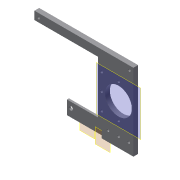
# Autodesk Inventor part: 01_Zeiss_Axiotech_adapterplate_left
Saved by Autodesk Inventor 2019 (Build 230136000, 136)
## iProperties
Created: 2019-05-02
Part Number: 01_Zeiss_Axiotech_adapterplate_left
Material: Generic
Document SubType Name: Modeling
Designer: diederichbenedict
Density: 1 g/cm^3
Appearance: Default
Author: diederichbenedict
Autodesk Inventor part; units mm, degrees
ref_plane "YZ Plane" through (0, 0, 0) normal (1, 0, 0) x (0, 1, 0)
ref_plane "XZ Plane" through (0, 0, 0) normal (0, 1, 0) x (-1, 0, 0)
ref_plane "Work Plane4" through (0, 0, 4) normal (0, 0, 1) x (1, 0, 0)
ref_plane "Work Plane5" through (25.4178, -3.2164, 6.83) normal (0, 0, 1) x (1, 0, 0)
ref_plane "Work Plane6" through (51, 60, 11) normal (0, 0, -1) x (0, 1, 0)
sketch "Sketch9" plane through (51, 60, 11) normal (0, 0, -1) x (0, 1, 0)
  circle A0 centre (0, 25) radius 1.95 construction
  circle A1 centre (-25, 0) radius 1.95 construction
  circle A2 centre (-25, -25) radius 1.95 construction
  circle A3 centre (25, 25) radius 1.95 construction
  circle A4 centre (25, -25) radius 1.95 construction
  circle A5 centre (-25, 25) radius 1.95 construction
  circle A6 centre (25, 0) radius 1.95 construction
  circle A7 centre (0, -25) radius 1.95 construction
  line L0 (-28, 30) -> (-30, 28) construction
  line L1 (-30, 28) -> (-30, -28) construction
  line L2 (-30, -28) -> (-28, -30) construction
  line L3 (-28, -30) -> (28, -30) construction
  line L4 (28, -30) -> (30, -28) construction
  line L5 (30, -28) -> (30, 28) construction
  line L6 (30, 28) -> (28, 30) construction
  line L7 (28, 30) -> (-28, 30) construction
  circle A8 centre (47.5, -118) radius 1.95 construction
  circle A9 centre (47.5, 16) radius 1.95 construction
  line L8 (53.5, -124) -> (41.5, -124)
  line L9 (41.5, -124) -> (41.5, 22)
  line L10 (41.5, 22) -> (53.5, 22)
  line L11 (53.5, 22) -> (53.5, -124)
  circle A10 centre (-60, -51) radius 15 projected
  line L12 (41.5, 22) -> (-60, 22)
  line L13 (-60, 22) -> (-60, -30)
  line L14 (-60, -30) -> (41.5, -30)
  line L15 (41.5, -30) -> (41.5, 22)
  circle A11 centre (47.5, -118) radius 1.95
  circle A12 centre (47.5, 16) radius 1.95
  circle A13 centre (25, -25) radius 2.25
  circle A14 centre (0, -25) radius 2.25
  circle A15 centre (-25, -25) radius 2.25
  circle A16 centre (-25, 0) radius 2.25
  circle A17 centre (25, 0) radius 2.25
  circle A18 centre (0, 0) radius 19.7399
  line L16 (-60, -30) -> (-40, -30)
  line L17 (-40, -30) -> (-40, -80)
  line L18 (-40, -80) -> (-60, -80)
  line L19 (-60, -80) -> (-60, -30)
  point P0 (-60, -51)
  dimension "d32" = 6
  dimension "d33" = 6
  dimension "d34" = 6
  dimension "d35" = 6
  dimension "d36" = 4.5
  dimension "d37" = 4.5
  dimension "d38" = 4.5
  dimension "d39" = 4.5
  dimension "d40" = 4.5
  dimension "d51" = 20
  dimension "d52" = 50
  constraints: 24 end point, 8 centre point, 6 coincident, 6 parallel, 3 horizontal, 3 perpendicular, 2 concentric, 1 point on line
  measures "d32" distance from line of A8.centre L8
  measures "d33" distance from line of L10 A9.centre
  measures "d34" distance from line of L11 A9.centre
  measures "d35" distance from line of L15 A9.centre
  measures "d36" diameter of A13
  measures "d37" diameter of A14
  measures "d38" diameter of A15
  measures "d39" diameter of A16
  measures "d40" diameter of A17
  measures "d51" distance of L17.end L18.end
  measures "d52" distance of L16.end L17.end
extrude "Extrusion8" add sketch "Sketch9" along normal blind 7 contours L8 L9 L10 L11 | L14 L13 L12 L9 | L17 L18 L19 A10 L14 | A10 L19 | A11 | A12 | A13 | A14 | A15 | A16 | A17 picked at (-54.0128, -49.762)
sketch "Sketch10" plane through (51, 60, 4) normal (0, 0, -1) x (-1, 0, 0)
  circle A0 centre (118, 47.5) radius 1.95 projected
  circle A1 centre (-16, 47.5) radius 1.95 projected
  circle A2 centre (-25, 0) radius 1.95 projected
  circle A3 centre (0, -25) radius 1.95 projected
  circle A4 centre (25, -25) radius 1.95 projected
  circle A5 centre (-25, 25) radius 1.95 projected
  circle A6 centre (25, 25) radius 1.95 projected
  circle A7 centre (-25, -25) radius 1.95 projected
  circle A8 centre (0, 25) radius 1.95 projected
  circle A9 centre (25, 0) radius 1.95 projected
  line L0 (-30, -28) -> (-28, -30) projected
  line L1 (-30, 28) -> (-30, -28) projected
  line L2 (-28, 30) -> (-30, 28) projected
  line L3 (28, 30) -> (-28, 30) projected
  line L4 (30, 28) -> (28, 30) projected
  line L5 (30, -28) -> (30, 28) projected
  line L6 (28, -30) -> (30, -28) projected
  line L7 (-28, -30) -> (28, -30) projected
  circle A10 centre (0, 0) radius 19.7399 construction
  line L8 (-22, -60) -> (80, -60) construction
  line L9 (80, -60) -> (80, -40) construction
  line L10 (80, -40) -> (30, -40) construction
  line L11 (30, -40) -> (30, 41.5) construction
  line L12 (30, 41.5) -> (124, 41.5) construction
  line L13 (124, 41.5) -> (124, 53.5) construction
  line L14 (124, 53.5) -> (-22, 53.5) construction
  line L15 (-22, 53.5) -> (-22, -60) construction
  line L16 (-15, -75) -> (15, -75) construction
  line L17 (15, -75) -> (15, -45) construction
  line L18 (15, -45) -> (-15, -45) construction
  line L19 (-15, -45) -> (-15, -75) construction
  line L20 (-22, -60) -> (80, -60) construction
  line L21 (-15, -75) -> (15, -45) construction
  line L22 (15, -75) -> (-15, -45) construction
  point P0 (51, -60)
  point P1 (0, -60)
  point P2 (0, -45)
  point P3 (15.5154, -45.1897)
  dimension "d53" = 30
  dimension "d54" = 30
  constraints: 12 end point, 3 midpoint, 2 parallel, 1 horizontal, 1 perpendicular, 1 point on line
  measures "d53" distance of L18.end L17.end
  measures "d54" distance of L17.end L16.end
hole "Hole2" at (-67, 107.5, 4) at (67, 107.5, 4) at (26, 85, 4) at (26, 60, 4) at (51, 85, 4) at (51, 35, 4) at (26, 35, 4) at (35.4846, 14.8103, 4) at (51, 15, 4) at (66, 15, 4) direction (0, 0, 1) diameter 3.9 depth 10 tip angle 118 counterbore diameter 8 counterbore depth 5
sketch "Sketch11" plane through (51, 60, 11) normal (0, 0, 1) x (1, 0, 0)
  line L0 (-41.7519, -83.7) -> (-44.35, -83.7) construction
  line L1 (-44.35, -83.7) -> (-44.35, -82.1) construction
  line L2 (-44.35, -82.1) -> (-57.05, -82.1) construction
  line L3 (-57.05, -82.1) -> (-57.05, -85.2) construction
  line L4 (-58.05, -85.2) -> (-57.05, -85.2) construction
  line L5 (-58.05, -85.2) -> (-58.05, -78.3) construction
  line L6 (-58.05, -78.3) -> (-71.65, -78.3) construction
  line L7 (-71.65, -78.3) -> (-71.65, -85.2) construction
  line L8 (-73.85, -85.2) -> (-71.65, -85.2) construction
  line L9 (-73.85, -85.2) -> (-73.85, -76.65) construction
  line L10 (-73.85, -76.65) -> (-70.5, -76.65) construction
  line L11 (-70.5, -76.65) -> (-70.5, -68.05) construction
  line L12 (-70.5, -68.05) -> (-75.5, -68.05) construction
  line L13 (-75.5, -68.05) -> (-75.5, -72.2) construction
  line L14 (-78.25, -72.2) -> (-75.5, -72.2) construction
  arc A0 (-79.7079, -54) -> (-78.25, -72.2) centre (-56.7997, -61.3233) ccw construction
  line L15 (-79.7079, -54) -> (-74.7, -54) construction
  line L16 (-74.7, -54) -> (-74.7, -58.75) construction
  line L17 (-74.7, -58.75) -> (-77.9, -58.75) construction
  arc A1 (-77.9, -58.75) -> (-78.9, -59.75) centre (-77.9, -59.75) ccw construction
  line L18 (-78.9, -59.75) -> (-78.9, -66.25) construction
  arc A2 (-78.9, -66.25) -> (-77.9, -67.25) centre (-77.9, -66.25) ccw construction
  line L19 (-77.9, -67.25) -> (-77.9, -68.75) construction
  line L20 (-77.9, -68.75) -> (-76.4, -68.75) construction
  line L21 (-76.4, -68.75) -> (-76.4, -67.25) construction
  line L22 (-76.4, -67.25) -> (-69.9, -67.25) construction
  line L23 (-69.9, -67.25) -> (-68.9, -68.25) construction
  line L24 (-68.9, -68.25) -> (-68.9, -76.7) construction
  line L25 (-68.9, -76.7) -> (-53.85, -76.7) construction
  arc A3 (-51.4, -79.15) -> (-53.85, -76.7) centre (-53.85, -79.15) ccw construction
  line L26 (-51.4, -79.15) -> (-51.4, -80.4) construction
  arc A4 (-51.4, -80.4) -> (-50.9, -80.9) centre (-50.9, -80.4) ccw construction
  line L27 (-50.9, -80.9) -> (-44.9, -80.9) construction
  arc A5 (-44.9, -80.9) -> (-43.9, -79.9) centre (-44.9, -79.9) ccw construction
  line L28 (-43.9, -79.9) -> (-43.9, -78.3) construction
  line L29 (-43.9, -78.3) -> (-49.9, -78.3) construction
  arc A6 (-50.9, -77.3) -> (-49.9, -78.3) centre (-49.9, -77.3) ccw construction
  line L30 (-50.9, -77.3) -> (-50.9, -76.2) construction
  arc A7 (-50.9, -76.2) -> (-52.9, -74.2) centre (-52.9, -76.2) ccw construction
  line L31 (-52.9, -74.2) -> (-68.5, -74.2) construction
  line L32 (-68.5, -74.2) -> (-68.5, -65.95) construction
  line L33 (-68.5, -65.95) -> (-69.95, -64.5) construction
  line L34 (-69.95, -64.5) -> (-78.5, -64.5) construction
  line L35 (-78.5, -64.5) -> (-78.5, -62.5) construction
  line L36 (-78.5, -62.5) -> (-74.5, -62.5) construction
  line L37 (-74.5, -62.5) -> (-74.5, -50.95) construction
  line L38 (-74.5, -50.95) -> (-71, -50.95) construction
  line L39 (-71, -50.95) -> (-70, -49.95) construction
  line L40 (-70, -45) -> (-70, -49.95) construction
  line L41 (-70, -45) -> (-54.55, -45) construction
  line L42 (-54.55, -45) -> (-54.55, -35.2) construction
  line L43 (-45.55, -35.2) -> (-54.55, -35.2) construction
  line L44 (-40.55, -38.0868) -> (-45.55, -35.2) construction
  line L45 (-40.55, -40.2) -> (-40.55, -38.0868) construction
  line L46 (-38.55, -40.2) -> (-40.55, -40.2) construction
  line L47 (-38.55, -40.2) -> (-38.55, -56.2) construction
  line L48 (-38.55, -56.2) -> (-28.25, -56.2) construction
  line L49 (-28.25, -56.2) -> (-28.25, -59.4) construction
  line L50 (-28.25, -59.4) -> (-40.45, -59.4) construction
  line L51 (-40.45, -59.4) -> (-40.45, -59.9) construction
  line L52 (-40.45, -59.9) -> (-37.45, -60.9) construction
  line L53 (-37.45, -60.9) -> (-31.75, -60.9) construction
  line L54 (-31.75, -60.9) -> (-31.75, -63.9) construction
  line L55 (-31.75, -63.9) -> (-36.75, -63.9) construction
  line L56 (-36.75, -63.9) -> (-36.75, -64.9) construction
  arc A8 (-36.75, -64.9) -> (-40.55, -70) centre (-32.7635, -71.836) ccw construction
  line L57 (-40.55, -83.0061) -> (-40.55, -70) construction
  line L58 (-41.7519, -83.7) -> (-40.55, -83.0061) construction
  line L59 (-37.75, -62.9) -> (-32.75, -62.9) construction
  line L60 (-32.75, -62.9) -> (-32.75, -61.9) construction
  line L61 (-32.75, -61.9) -> (-37.6123, -61.9) construction
  line L62 (-37.6123, -61.9) -> (-40.45, -60.9541) construction
  line L63 (-40.45, -60.9541) -> (-40.45, -67.1543) construction
  arc A9 (-37.75, -64.3437) -> (-40.45, -67.1543) centre (-32.7635, -71.836) ccw construction
  line L64 (-37.75, -64.3437) -> (-37.75, -62.9) construction
  circle A10 centre (-53.85, -79.15) radius 1.45 construction
  arc A11 (-65.475, -56.2) -> (-64.475, -57.2) centre (-64.475, -56.2) ccw construction
  line L65 (-64.475, -57.2) -> (-63.025, -57.2) construction
  line L66 (-63.025, -57.2) -> (-63.025, -68.2) construction
  line L67 (-63.025, -68.2) -> (-45.725, -68.2) construction
  arc A12 (-45.725, -68.2) -> (-44.725, -67.2) centre (-45.725, -67.2) ccw construction
  line L68 (-44.725, -67.2) -> (-44.725, -64.7) construction
  arc A13 (-44.725, -64.7) -> (-45.725, -63.7) centre (-45.725, -64.7) ccw construction
  line L69 (-45.725, -63.7) -> (-47.225, -63.7) construction
  line L70 (-47.225, -63.7) -> (-47.225, -53) construction
  line L71 (-47.225, -53) -> (-64.475, -53) construction
  arc A14 (-64.475, -53) -> (-65.475, -54) centre (-64.475, -54) ccw construction
  line L72 (-65.475, -54) -> (-65.475, -56.2) construction
  arc A15 (-75.5, -46.2) -> (-79.7079, -54) centre (-56.7997, -61.3233) ccw construction
  line L73 (-70, -46.2) -> (-75.5, -46.2) construction
  line L74 (-70, -49.95) -> (-70, -46.2) construction
  line L75 (-71, -50.95) -> (-70, -49.95) construction
  line L76 (-74.5, -50.95) -> (-71, -50.95) construction
  line L77 (-74.5, -54) -> (-74.5, -50.95) construction
  line L78 (-79.7079, -54) -> (-74.5, -54) construction
  circle A16 centre (-74.4691, -48.3) radius 0.9 construction
  circle A17 centre (-27.75, -65) radius 0.9 construction
  line L79 (-28.25, -59.4) -> (-40.45, -59.4) construction
  line L80 (-28.25, -57.9) -> (-28.25, -59.4) construction
  line L81 (-25.75, -57.9) -> (-28.25, -57.9) construction
  line L82 (-25.75, -67) -> (-25.75, -57.9) construction
  line L83 (-32.55, -67) -> (-25.75, -67) construction
  arc A18 (-32.55, -67) -> (-40.55, -75) centre (-32.55, -75) ccw construction
  line L84 (-40.55, -70) -> (-40.55, -75) construction
  arc A19 (-36.75, -64.9) -> (-40.55, -70) centre (-32.7635, -71.836) ccw construction
  line L85 (-36.75, -63.9) -> (-36.75, -64.9) construction
  line L86 (-31.75, -63.9) -> (-36.75, -63.9) construction
  line L87 (-31.75, -60.9) -> (-31.75, -63.9) construction
  line L88 (-37.45, -60.9) -> (-31.75, -60.9) construction
  line L89 (-40.45, -59.9) -> (-37.45, -60.9) construction
  line L90 (-40.45, -59.4) -> (-40.45, -59.9) construction
  circle A20 centre (0, -45) radius 1.95 construction
  circle A21 centre (-25, -25) radius 1.95 construction
  circle A22 centre (0, 25) radius 1.95 construction
  circle A23 centre (-25, 25) radius 1.95 construction
  circle A24 centre (-118, 47.5) radius 1.95 construction
  circle A25 centre (16, 47.5) radius 1.95 construction
  circle A26 centre (-25, 0) radius 1.95 construction
  circle A27 centre (0, -25) radius 1.95 construction
  circle A28 centre (-15.5154, -45.1897) radius 1.95 construction
  circle A29 centre (15, -45) radius 1.95 construction
  circle A30 centre (0, 0) radius 19.7399 construction
  line L91 (-124, 53.5) -> (22, 53.5) construction
  line L92 (-124, 41.5) -> (-124, 53.5) construction
  line L93 (-30, 41.5) -> (-124, 41.5) construction
  line L94 (-30, -40) -> (-30, 41.5) construction
  line L95 (-80, -40) -> (-30, -40) construction
  line L96 (-80, -60) -> (-80, -40) construction
  line L97 (22, -60) -> (-80, -60) construction
  line L98 (22, 53.5) -> (22, -60) construction
  line L99 (-80, -40) -> (-30, -40) projected
  line L100 (22, -60) -> (-80, -60) projected
  line L101 (-80, -40) -> (-25, -40)
  line L102 (-25, -40) -> (-25, -60)
  line L103 (-25, -60) -> (-80, -60)
  line L104 (-80, -60) -> (-80, -40)
  point P0 (-51, -60)
  constraints: 8 end point, 2 parallel, 1 horizontal, 1 perpendicular, 1 point on line
extrude "Extrusion9" cut sketch "Sketch11" against normal blind 4
sketch "Sketch12" plane through (51, 60, 7) normal (0, 0, 1) x (1, 0, 0)
  circle A0 centre (-74.4691, -48.3) radius 0.9 projected
  circle A1 centre (-74.4691, -48.3) radius 2
  point P0 (-51, -60)
  dimension "d57" = 4
  constraints: 1 centre point, 1 coincident
  measures "d57" diameter of A1
ref_plane "Work Plane7" through (-86.9, -137.5, 4) normal (0, 0, 1) x (1, 0, 0)
extrude "Extrusion10" add sketch "Sketch12" against normal up to surface (3 mm away)
sketch "Sketch13" plane through (51, 60, 4) normal (0, 0, -1) x (-1, 0, 0)
  circle A0 centre (74.4691, -48.3) radius 0.9 projected
  point P0 (51, -60)
hole "Hole3" at (-23.4691, 11.7, 4) direction (0, 0, 1) diameter 2 depth 10 tip angle 118 counterbore diameter 6 counterbore depth 3
shell "Shell2" thickness 2 removed faces 1 at (7, 108.0892, 4)
body "Solid2"
